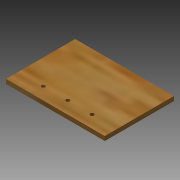
# Autodesk Inventor part: segment0a
Saved by Autodesk Inventor 2013 (Build 170138000, 138)
## iProperties
Created: 2014-10-12
Part Number: segment0a
Material: Plywood, Finish
Document SubType Name: Modeling
Designer: Masta
Density: 1 g/cm^3
Author: Masta
Autodesk Inventor part; units mm, degrees
ref_plane "YZ Plane" through (0, 0, 0) normal (1, 0, 0) x (0, 1, 0)
ref_plane "XZ Plane" through (0, 0, 0) normal (0, 1, 0) x (-1, 0, 0)
ref_plane "XY Plane" through (0, 0, 0) normal (0, 0, 1) x (1, 0, 0)
sketch "Sketch1" plane through (0, 0, 0) normal (0, 0, 1) x (1, 0, 0)
  line L0 (0, 0) -> (0, 40)
  line L1 (0, 40) -> (0, 46)
  line L2 (0, 46) -> (40, 46)
  line L3 (40, -10) -> (0, -10)
  line L4 (0, -10) -> (0, 0)
  line L5 (40, 46) -> (40, 40)
  line L6 (40, 40) -> (40, -10)
  line L7 (0, 40) -> (40, 40) construction
  line L8 (0, 0) -> (19.75, 0) construction
  dimension "d0" = 40
  dimension "d1" = 6
  dimension "d2" = 10
  dimension "d3" = 40
  dimension "d4" = 40
  dimension "d5" = 19.75
  constraints: 18 end point, 4 parallel, 2 perpendicular, 1 coincident, 1 collinear, 1 vertical
  measures "d0" distance of L0.start L0.end
  measures "d1" distance of L0.end L1.end
  measures "d2" distance of L0.start L3.end
  measures "d3" distance of L3.start L3.end
  measures "d4" distance of L1.end L2.end
  measures "d5" distance of L0.start L8.end
extrude "Extrusion1" add sketch "Sketch1" along normal blind 3.5
fillet "Fillet1" [suppressed]
hole "Hole1" at (0, 0, 0) at (19.75, 0, 0) direction (0, 0, 1) diameter 3 end through all
mirror "Mirror1" about plane through (0, 40, 0) normal (-1, 0, 0)
body "Solid1"
